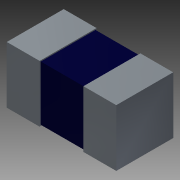
# Autodesk Inventor part: 0402_res
Saved by Autodesk Inventor 2013 (Build 170138000, 138)
## iProperties
Created: 2015-06-30
Part Number: 0402_res
Material: Ogólny
Document SubType Name: Modeling
Designer: terg
Density: 1 g/cm^3
Author: terg
Autodesk Inventor part; units mm, degrees
ref_plane "YZ Plane" through (0, 0, 0) normal (1, 0, 0) x (0, 1, 0)
ref_plane "XZ Plane" through (0, 0, 0) normal (0, 1, 0) x (-1, 0, 0)
ref_plane "XY Plane" through (0, 0, 0) normal (0, 0, 1) x (1, 0, 0)
sketch "Szkic1" plane through (0, 0, 0) normal (0, 1, 0) x (-1, 0, 0)
  line L0 (0, 0) -> (1, 0)
  line L1 (1, 0) -> (1, 0.5)
  line L2 (1, 0.5) -> (0, 0.5)
  line L3 (0, 0.5) -> (0, 0)
  dimension "d0" = 1
  dimension "d1" = 0.5
  constraints: 8 end point, 2 parallel, 1 horizontal, 1 perpendicular
  measures "d0" distance of L2.end L1.end
  measures "d1" distance of L1.end L0.end
extrude "Wyciągnięcie proste1" add sketch "Szkic1" along normal blind 0.5
sketch "Szkic2" plane through (0, 0.5, 0) normal (0, 1, 0) x (1, 0, 0)
  line L0 (-1, 0) -> (-0.7, 0)
  line L1 (-0.7, 0) -> (-0.7, -0.5)
  line L2 (-0.7, -0.5) -> (-1, -0.5)
  line L3 (-1, -0.5) -> (-1, 0)
  line L4 (0, 0) -> (-0.3, 0)
  line L5 (-0.3, 0) -> (-0.3, -0.5)
  line L6 (-0.3, -0.5) -> (0, -0.5)
  line L7 (0, -0.5) -> (0, 0)
  dimension "d4" = 0.3
  dimension "d5" = 0.5
  dimension "d6" = 0.3
  dimension "d7" = 0.5
  constraints: 16 end point, 4 parallel, 2 horizontal, 2 perpendicular
  measures "d4" distance of L1.end L2.end
  measures "d5" distance of L0.end L1.end
  measures "d6" distance of L6.end L5.end
  measures "d7" distance of L5.end L4.end
extrude "Wyciągnięcie proste2" add sketch "Szkic2" along normal blind 0.01 and the other way blind 0.51
sketch "Szkic4" plane through (-0.7, 0, 0.5) normal (0, 0, 1) x (1, 0, 0)
  line L0 (-0.3, -0.01) -> (-0.3, 0.51) projected
  line L1 (0, -0.01) -> (-0.3, -0.01) projected
  line L2 (-0.3, 0.51) -> (0, 0.51)
  line L3 (0, 0.51) -> (0, -0.01)
  line L4 (0, -0.01) -> (-0.3, -0.01)
  line L5 (-0.3, -0.01) -> (-0.3, 0.51)
  line L6 (0.7, 0.51) -> (0.4, 0.51)
  line L7 (0.4, 0.51) -> (0.4, -0.01)
  line L8 (0.4, -0.01) -> (0.7, -0.01)
  line L9 (0.7, -0.01) -> (0.7, 0.51)
  point P0 (0.7, 0)
  constraints: 16 end point, 4 parallel, 2 horizontal, 2 perpendicular
extrude "Wyciągnięcie proste3" add sketch "Szkic4" along normal blind 0.01 and the other way blind 0.51
